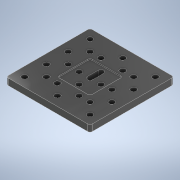
# Autodesk Inventor part: piezamovil
Saved by Autodesk Inventor 2022 (Build 260153000, 153)
## iProperties
Created: 2022-03-21
Part Number: piezamovil
Material: Generic
Document SubType Name: Modeling
Designer: ferna
Density: 1 g/cm^3
Appearance: Dark Gray
Mass: 37.654 g
Surface Area: 168.371 cm^2
Volume: 37.654 cm^3
Author: ferna
Autodesk Inventor part; units mm, degrees
ref_plane "YZ Plane" through (0, 0, 0) normal (1, 0, 0) x (0, 1, 0)
ref_plane "XZ Plane" through (0, 0, 0) normal (0, 1, 0) x (-1, 0, 0)
ref_plane "XY Plane" through (0, 0, 0) normal (0, 0, 1) x (1, 0, 0)
sketch "Sketch1" plane through (0, 0, 0) normal (0, 1, 0) x (-1, 0, 0)
  line L0 (0, 0) -> (75, 0)
  line L1 (77, -2) -> (77, -75)
  line L2 (75, -77) -> (2, -77)
  line L3 (0, -75) -> (0, 0)
  line L4 (0, 0) -> (0, -8.5)
  line L5 (6, -8.5) -> (8.5, -8.5)
  line L6 (8.5, -48.5) -> (8.5, -68.5)
  circle A0 centre (8.5, -8.5) radius 2.5
  circle A1 centre (8.5, -28.5) radius 2.5
  circle A2 centre (8.5, -48.5) radius 2.5
  circle A3 centre (8.5, -68.5) radius 2.5
  line L7 (68.5, -28.5) -> (68.5, -48.5)
  line L8 (68.5, -48.5) -> (68.5, -68.5)
  line L9 (68.5, -68.5) -> (38.5, -68.5)
  circle A4 centre (38.5, -8.5) radius 2.5
  circle A5 centre (68.5, -8.5) radius 2.5
  circle A6 centre (68.5, -28.5) radius 2.5
  circle A7 centre (68.5, -48.5) radius 2.5
  circle A8 centre (68.5, -68.5) radius 2.5
  circle A9 centre (38.5, -68.5) radius 2.5
  line L10 (77, 0) -> (58.5, 0)
  line L11 (58.5, -18.5) -> (61, -18.5)
  line L12 (77, -18.5) -> (77, 0)
  line L13 (2, 0) -> (18.5, 0)
  line L14 (18.5, -8.5) -> (18.5, -18.5)
  line L15 (18.5, -18.5) -> (0, -18.5)
  line L16 (0, -18.5) -> (0, -2)
  line L17 (0, -77) -> (18.5, -77)
  line L18 (18.5, -61) -> (18.5, -58.5)
  line L19 (0, -58.5) -> (0, -77)
  circle A10 centre (58.5, -18.5) radius 2.5
  circle A11 centre (18.5, -18.5) radius 2.5
  circle A12 centre (18.5, -58.5) radius 2.5
  circle A13 centre (58.5, -58.5) radius 2.5
  line L20 (18.5, -18.5) -> (28.5, -18.5)
  line L21 (58.5, -58.5) -> (48.5, -58.5)
  circle A14 centre (28.5, -18.5) radius 2.5
  circle A15 centre (48.5, -18.5) radius 2.5
  circle A16 centre (48.5, -58.5) radius 2.5
  circle A17 centre (28.5, -58.5) radius 2.5
  line L22 (58.5, -38.5) -> (48.5, -38.5)
  line L23 (28.5, -38.5) -> (18.5, -38.5)
  circle A18 centre (58.5, -38.5) radius 2.5
  circle A19 centre (48.5, -38.5) radius 2.5
  circle A20 centre (28.5, -38.5) radius 2.5
  circle A21 centre (18.5, -38.5) radius 2.5
  circle A22 centre (38.5, -28.5) radius 2.5
  circle A23 centre (38.5, -38.5) radius 2.5
  line L24 (28.5, -58.5) -> (28.5, -38.5)
  circle A24 centre (38.5, -48.5) radius 2.5
  line L25 (36, -48.5) -> (36, -38.5)
  line L26 (41, -38.5) -> (41, -48.5)
  arc A25 (77, -2) -> (75, 0) centre (75, -2) ccw
  arc A26 (75, -77) -> (77, -75) centre (75, -75) ccw
  arc A27 (0, -75) -> (2, -77) centre (2, -75) ccw
  arc A28 (2, 0) -> (0, -2) centre (2, -2) ccw
  line L27 (68.5, -8.5) -> (68.5, -11)
  line L28 (68.5, -26) -> (68.5, -28.5)
  line L29 (58.5, 0) -> (58.5, -8.5)
  line L30 (58.5, -16) -> (58.5, -18.5)
  line L31 (38.5, -8.5) -> (41, -8.5)
  line L32 (66, -8.5) -> (68.5, -8.5)
  line L33 (58.5, -18.5) -> (58.5, -21)
  line L34 (58.5, -36) -> (58.5, -38.5)
  line L35 (58.5, -18.5) -> (56, -18.5)
  line L36 (51, -18.5) -> (48.5, -18.5)
  line L37 (48.5, -18.5) -> (46.7322, -20.2678)
  line L38 (40.2678, -26.7322) -> (28.5, -38.5)
  line L39 (28.5, -18.5) -> (40.2678, -30.2678)
  line L40 (46.7322, -36.7322) -> (48.5, -38.5)
  line L41 (48.5, -38.5) -> (46, -38.5)
  line L42 (41, -38.5) -> (28.5, -38.5)
  line L43 (48.5, -38.5) -> (46.7322, -40.2678)
  line L44 (41, -46) -> (36.7322, -50.2678)
  line L45 (30.2678, -56.7322) -> (28.5, -58.5)
  line L46 (48.5, -58.5) -> (36, -46)
  line L47 (30.2678, -40.2678) -> (28.5, -38.5)
  line L48 (18.5, -58.5) -> (21, -58.5)
  line L49 (26, -58.5) -> (28.5, -58.5)
  line L50 (18.5, -58.5) -> (16, -58.5)
  line L51 (8.5, -58.5) -> (0, -58.5)
  line L52 (8.5, -28.5) -> (8.5, -31)
  line L53 (8.5, -46) -> (8.5, -48.5)
  line L54 (8.5, -8.5) -> (8.5, -11)
  line L55 (8.5, -26) -> (8.5, -28.5)
  line L56 (8.5, -8.5) -> (11, -8.5)
  line L57 (18.5, -8.5) -> (38.5, -8.5)
  line L58 (28.5, -38.5) -> (28.5, -36)
  line L59 (28.5, -21) -> (28.5, -18.5)
  point P0 (77, -77)
  dimension "d9" = 5
  dimension "d15" = 5
  dimension "d17" = 5
  dimension "d29" = 5
  dimension "d32" = 5
  dimension "d0" = 77
  dimension "d1" = 77
  dimension "d2" = 8.5
  dimension "d3" = 8.5
  dimension "d4" = 20
  dimension "d5" = 20
  dimension "d6" = 20
  dimension "d7" = 5
  dimension "d8" = 5
  dimension "d10" = 5
  dimension "d11" = 30
  dimension "d12" = 30
  dimension "d13" = 20
  dimension "d14" = 20
  dimension "d16" = 5
  dimension "d18" = 18.5
  dimension "d19" = 18.5
  dimension "d20" = 18.5
  dimension "d21" = 18.5
  dimension "d22" = 18.5
  dimension "d23" = 18.5
  dimension "d24" = 5
  dimension "d25" = 5
  dimension "d26" = 10
  dimension "d27" = 10
  dimension "d28" = 10
  dimension "d30" = 5
  dimension "d31" = 20
  dimension "d33" = 5
  dimension "d34" = 5
  dimension "d35" = 2
  dimension "d36" = 2
  constraints: 120 end point, 38 point on circle, 30 perpendicular, 24 centre point, 21 coincident, 17 point on line, 14 parallel, 9 horizontal, 9 tangent, 4 vertical, 4 vertical alignment, 2 equal radius, 1 horizontal alignment, 1 midpoint, 10 other
  measures "d0" distance of point (77, -77) L17.start
  measures "d1" distance of L10.start point (77, -77)
  measures "d2" distance of L0.start L4.end
  measures "d3" distance of L4.end L5.end
  measures "d4" distance of L5.end L52.start
  measures "d5" distance of L52.start L6.start
  measures "d6" distance of L6.start L6.end
  measures "d7" diameter of A0
  measures "d8" diameter of A1
  measures "d10" diameter of A3
  measures "d11" distance of L56.start L31.start
  measures "d12" distance of L31.start L27.start
  measures "d13" distance of L27.start L7.start
  measures "d14" distance of L7.start L7.end
  measures "d16" diameter of A5
  measures "d18" distance of L12.start L11.start
  measures "d19" distance of L11.start L10.end
  measures "d20" distance of L14.end L15.end
  measures "d21" distance of L13.end L14.end
  measures "d22" distance of L19.start L18.end
  measures "d23" distance of L18.end L17.end
  measures "d24" diameter of A10
  measures "d25" diameter of A12
  measures "d26" distance of L33.start L36.end
  measures "d27" distance of L20.start L20.end
  measures "d28" distance of L21.start L21.end
  measures "d30" diameter of A15
  measures "d31" distance of L33.start L22.start
  measures "d33" diameter of A22
  measures "d34" diameter of A24
  measures "d35" radius of A25
  measures "d36" radius of A26
extrude "Extrusion1" add sketch "Sketch1" along normal blind 6 contours L0 A25 L1 A26 L2 A27 L3 A28
sketch "Sketch2" plane through (0, 6, 0) normal (0, 1, 0) x (1, 0, 0)
  line L0 (0, 0) -> (-23.5, 0)
  line L1 (-23.5, 0) -> (-23.5, 23.5)
  line L2 (-23.5, 23.5) -> (0, 23.5)
  line L3 (0, 23.5) -> (0, 0)
  line L4 (-77, 75) -> (-77, 2) projected
  line L5 (-77, 67.2397) -> (-77, 80.0778)
  line L6 (-2, 77) -> (-75, 77) projected
  line L7 (-67.8517, 77) -> (-77, 77)
  line L8 (-77, 77) -> (-53.5, 77)
  line L9 (-53.5, 77) -> (-53.5, 53.5)
  line L10 (-53.5, 53.5) -> (-77, 53.5)
  line L11 (-77, 53.5) -> (-77, 77)
  line L12 (-51.5, 53.5) -> (-25.5, 53.5)
  line L13 (-23.5, 51.5) -> (-23.5, 25.5)
  line L14 (-25.5, 23.5) -> (-51.5, 23.5)
  line L15 (-53.5, 25.5) -> (-53.5, 51.5)
  arc A0 (-53.5, 25.5) -> (-51.5, 23.5) centre (-51.5, 25.5) ccw
  arc A1 (-25.5, 23.5) -> (-23.5, 25.5) centre (-25.5, 25.5) ccw
  arc A2 (-23.5, 51.5) -> (-25.5, 53.5) centre (-25.5, 51.5) ccw
  arc A3 (-51.5, 53.5) -> (-53.5, 51.5) centre (-51.5, 51.5) ccw
  dimension "d39" = 23.5
  dimension "d40" = 23.5
  dimension "d41" = 23.5
  dimension "d42" = 23.5
  dimension "d43" = 2
  constraints: 28 end point, 8 point on circle, 8 tangent, 7 point on line, 6 parallel, 4 centre point, 4 perpendicular, 3 equal radius, 3 horizontal, 1 collinear
  measures "d39" distance of L1.end L2.end
  measures "d40" distance of L0.end L1.end
  measures "d41" distance of L9.end L10.end
  measures "d42" distance of L8.end L9.end
  measures "d43" radius of A0
extrude "Extrusion2" cut sketch "Sketch2" against normal blind 1 contours L12 A2 L13 A1 L14 A0 L15 A3
sketch "Sketch3" plane through (0, 0, 0) normal (0, -1, 0) x (1, 0, 0)
  line L0 (-51.5, -53.5) -> (-25.5, -53.5) projected
  line L1 (-53.5, -25.5) -> (-53.5, -51.5) projected
  line L2 (-25.5, -23.5) -> (-51.5, -23.5) projected
  line L3 (-23.5, -51.5) -> (-23.5, -25.5) projected
  line L4 (-53.5, -53.5) -> (-23.5, -53.5)
  line L5 (-23.5, -53.5) -> (-23.5, -38.5)
  line L6 (-53.5, -38.5) -> (-23.5, -38.5)
  line L7 (-53.5, -38.5) -> (-53.5, -53.5)
  point P0 (0, 0)
  constraints: 8 end point, 2 midpoint, 2 perpendicular, 1 point on line
extrude "Extrusion3" add sketch "Sketch3" along normal blind 15
sketch "Sketch4" plane through (-23.5, 0, -53.5) normal (0, 0, -1) x (-1, 0, 0)
  line L0 (2.5, 0) -> (0, 0) projected
  line L1 (0, 0) -> (0, -15) projected
  line L2 (0, -8) -> (15, -8)
  line L3 (30, 0) -> (30, -15) projected
  circle A0 centre (15, -8) radius 4
  line L4 (0, 0) -> (0, -15) projected
  line L5 (0, -8) -> (0, -15)
  line L6 (30, -15) -> (0, -15) projected
  point P0 (-23.5, 0)
  dimension "d49" = 15
  dimension "d50" = 8
  dimension "d53" = 7
  constraints: 4 end point, 1 centre point, 1 coincident, 1 collinear, 1 perpendicular, 1 point on line
  measures "d49" distance of L2.start L2.end
  measures "d50" diameter of A0
  measures "d53" distance between parallel lines of L6 L2
extrude "Extrusion4" cut sketch "Sketch4" against normal blind 22
sketch "Sketch5" plane through (0, 6, 0) normal (0, 1, 0) x (1, 0, 0)
  arc A0 (-25.5, 23.5) -> (-23.5, 25.5) centre (-25.5, 25.5) ccw projected
  line L0 (-25.5, 23.5) -> (-51.5, 23.5) projected
  arc A1 (-53.5, 25.5) -> (-51.5, 23.5) centre (-51.5, 25.5) ccw projected
  line L1 (-53.5, 25.5) -> (-53.5, 51.5) projected
  arc A2 (-51.5, 53.5) -> (-53.5, 51.5) centre (-51.5, 51.5) ccw projected
  line L2 (-51.5, 53.5) -> (-25.5, 53.5) projected
  arc A3 (-23.5, 51.5) -> (-25.5, 53.5) centre (-25.5, 51.5) ccw projected
  line L3 (-23.5, 51.5) -> (-23.5, 25.5) projected
  arc A4 (0, 75) -> (-2, 77) centre (-2, 75) ccw projected
  line L4 (-2, 77) -> (-75, 77) projected
  arc A5 (-75, 77) -> (-77, 75) centre (-75, 75) ccw projected
  line L5 (-77, 75) -> (-77, 2) projected
  arc A6 (-77, 2) -> (-75, 0) centre (-75, 2) ccw projected
  line L6 (-75, 0) -> (-2, 0) projected
  arc A7 (-2, 0) -> (0, 2) centre (-2, 2) ccw projected
  line L7 (0, 2) -> (0, 75) projected
  circle A8 centre (-58.5, 38.5) radius 2.5 projected
  circle A9 centre (-68.5, 28.5) radius 2.5 projected
  circle A10 centre (-68.5, 48.5) radius 2.5 projected
  circle A11 centre (-68.5, 68.5) radius 2.5 projected
  circle A12 centre (-8.5, 48.5) radius 2.5 projected
  circle A13 centre (-8.5, 68.5) radius 2.5 projected
  circle A14 centre (-18.5, 38.5) radius 2.5 projected
  circle A15 centre (-28.5, 58.5) radius 2.5 projected
  circle A16 centre (-58.5, 58.5) radius 2.5 projected
  circle A17 centre (-48.5, 58.5) radius 2.5 projected
  circle A18 centre (-28.5, 18.5) radius 2.5 projected
  circle A19 centre (-38.5, 8.5) radius 2.5 projected
  circle A20 centre (-18.5, 18.5) radius 2.5 projected
  circle A21 centre (-18.5, 58.5) radius 2.5 projected
  circle A22 centre (-58.5, 18.5) radius 2.5 projected
  circle A23 centre (-8.5, 28.5) radius 2.5 projected
  circle A24 centre (-8.5, 8.5) radius 2.5 projected
  circle A25 centre (-68.5, 8.5) radius 2.5 projected
  circle A26 centre (-38.5, 68.5) radius 2.5 projected
  circle A27 centre (-48.5, 18.5) radius 2.5 projected
  point P0 (0, 0)
body "Solid1" dims "d19" = 18.5
